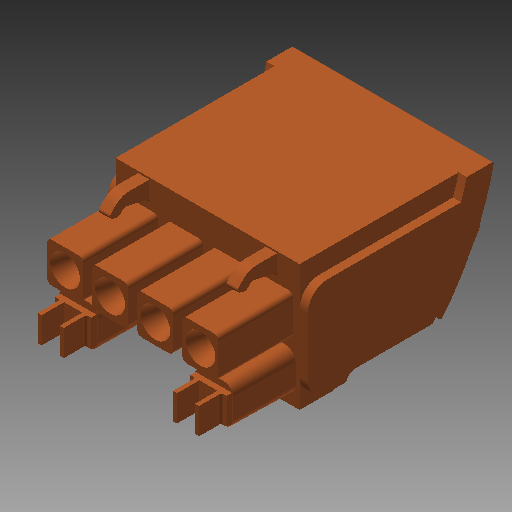
# Autodesk Inventor part: BHZ 5.00/04/90LH BK/OR 1063280000
Saved by Autodesk Inventor 2019.3 (Build 233278000, 278)
## iProperties
Category: PARTsolutions
Company: WEIDMUELLER
Created: 2018-11-15
Part Number: BHZ 5.00/04/90LH BK/OR 1063280000
Material: Generic
Catalog Web Link: www.cadenas.de
Description: BHZ 5.00/90LH-Electronics housings
Vendor: WEIDMUELLER
Document SubType Name: Modeling
Designer: psadmin
Manufacturer: WEIDMUELLER
Mass: 5.49278 g
Surface Area: 32.7214 cm^2
Volume: 5.49278 cm^3
Density: 1 g/cm^3
Appearance: PSOLRGB-219-112-51
PSOL_IDENT_0: {$CADENAS_DATA\23d-libs\weidmueller\elektronikgehaeuse\einbaugehaeuse\ch20m\zubehoer\bhz500_04_90_lh
PSOL_IDENT_1: .prj},213 {VTYP=3D},{NB=BHZ 5.00/04/90LH BK/OR 1063280000},{LINA=BHZ 5.00/04/90LH BK/OR 1063280000},
PSOL_IDENT_2: {NN=BHZ 5.00/90LH},{DATE=31.03.2017 09:22:38},{GEOMDATE=12.03.2014 15:03:00},{VERSION=},{LINEID=10},
PSOL_IDENT_3: {WBVAR=},{WBNUMERIC=}  {NB=BHZ 5.00/04/90LH BK/OR 1063280000},{LINA=BHZ 5.00/04/90LH BK/OR 106328000
PSOL_IDENT_4: 0},{KT=DUMMY},{BEST=1063280000},{BZ=BHZ 5.00/04/90LH BK/OR},{R=5.00},{P=4},{F=schwarz / orange},{FCO
PSOL_IDENT_5: DE=0.86,0.44,0.20,0.00}
NN: BHZ 5.00/90LH
NT: Electronics housings
NB: BHZ 5.00/04/90LH BK/OR 1063280000
NBSYN: $BZ. $BEST.
LINA: BHZ 5.00/04/90LH BK/OR 1063280000
BEST: 1063280000
BZ: BHZ 5.00/04/90LH BK/OR
R: 5
P: 4
F: black / orange
SUPPLIER: WEIDMUELLER
ARTICLENO: BHZ 5.00/04/90LH BK/OR 1063280000
BOMINFO: BHZ 5.00/04/90LH BK/OR 1063280000
CREATOR: CADENAS GmbH
Title: BHZ 5.00/04/90LH BK/OR 1063280000
Author: Cadenas PARTsolutions
Comments: Electronics housings
Autodesk Inventor part; units mm, degrees
sketch "Sketch_1" plane through (-3.6, 0, 0) normal (1, 0, 0) x (0, 0, -1)
  line L0 (0, 5.3) -> (0, -8.7)
  line L1 (0, -8.7) -> (3.6163, -8.7)
  arc A0 (3.6163, -8.7) -> (4.0993, -8.3294) centre (3.6163, -8.2) ccw
  line L2 (4.0993, -8.3294) -> (4.2837, -7.6412)
  arc A1 (5.2496, -6.9) -> (4.2837, -7.6412) centre (5.2496, -7.9) ccw
  line L3 (5.2496, -6.9) -> (13.7691, -6.9)
  arc A2 (13.7691, -6.9) -> (13.9423, -6.8) centre (13.7691, -6.7) ccw
  line L4 (13.9423, -6.8) -> (14.0722, -6.575)
  arc A3 (14.2021, -6.5) -> (14.0722, -6.575) centre (14.2021, -6.65) ccw
  line L5 (14.2021, -6.5) -> (14.2286, -6.5)
  arc A4 (14.4625, -6.635) -> (14.2286, -6.5) centre (14.2286, -6.77) ccw
  line L6 (14.4625, -6.635) -> (14.5371, -6.7642)
  arc A5 (14.5371, -6.7642) -> (14.9821, -6.7975) centre (14.7709, -6.6292) ccw
  arc A6 (14.9821, -6.7975) -> (17.8754, -2.4) centre (-7.6977, 11.2753) ccw
  line L7 (17.8754, -2.4) -> (19.05, -2.4)
  line L8 (19.05, -2.4) -> (19.05, -0.5176)
  arc A7 (19.2612, 0.588) -> (19.05, -0.5176) centre (22.05, -0.5176) ccw
  arc A8 (19.2612, 0.588) -> (20.6278, 5.0571) centre (-7.6977, 11.2753) ccw
  arc A9 (20.6278, 5.0571) -> (20.4324, 5.3) centre (20.4324, 5.1) ccw
  line L9 (20.4324, 5.3) -> (0, 5.3)
  constraints: 20 end point, 20 point on circle, 10 centre point
extrude "Extrusion1" add sketch "Sketch_1" along normal blind 22.2
sketch "Sketch_2" plane through (0, 0, -19.505) normal (0, 0, 1) x (1, 0, 0)
  line L0 (-5, 0.5) -> (20, 0.5)
  line L1 (-5, 0.4) -> (-5, -3)
  line L2 (-5, -3) -> (20, -3)
  line L3 (20, -3) -> (20, 0.45)
  line L4 (20, 0.45) -> (17.4, 0.45)
  line L5 (17.4, 0.45) -> (17.4, 0)
  arc A0 (13.2353, -1.6266) -> (17.4, 0) centre (15, 0) ccw
  arc A1 (13.2353, -1.6266) -> (11.7647, -1.6266) centre (12.5, -2.3043) ccw
  arc A2 (8.2353, -1.6266) -> (11.7647, -1.6266) centre (10, 0) ccw
  arc A3 (8.2353, -1.6266) -> (6.7647, -1.6266) centre (7.5, -2.3043) ccw
  arc A4 (3.2353, -1.6266) -> (6.7647, -1.6266) centre (5, 0) ccw
  arc A5 (3.2353, -1.6266) -> (1.7647, -1.6266) centre (2.5, -2.3043) ccw
  arc A6 (-2.4, 0) -> (1.7647, -1.6266) centre (0, 0) ccw
  line L6 (-2.4, 0) -> (-2.4, 0.4)
  line L7 (-2.4, 0.4) -> (-5, 0.4)
  constraints: 16 end point, 14 point on circle, 7 centre point
revolve "Revolution1" cut sketch "Sketch_2" angle 30 about axis through (-5, 0.5, -19.505) along (-1, 0, 0)
sketch "Sketch_5" plane through (0, 0, 0) normal (1, 0, 0) x (0, 1, 0)
  line L0 (0, -21) -> (0, -16)
  line L1 (0, -16) -> (1.9, -16)
  line L2 (1.9, -16) -> (1.9, -21)
  line L3 (1.9, -21) -> (0, -21)
  line L4 (0, -21) -> (0, -16)
  constraints: 10 end point
revolve "Revolution2" cut sketch "Sketch_5" angle 360 about axis through (0, 0, -21) along (0, 0, -1)
pattern_linear "Rectangular Pattern1" count 4 spacing 5 along (1, 0, 0) of "Revolution2"
sketch "Sketch_7" plane through (0, 0, 0) normal (0, 0, 1) x (1, 0, 0)
  line L0 (-2, 1.7) -> (-2, -1.7)
  arc A0 (-2, -1.7) -> (-1.5, -2.2) centre (-1.5, -1.7) ccw
  line L1 (-1.5, -2.2) -> (1.5, -2.2)
  arc A1 (1.5, -2.2) -> (2, -1.7) centre (1.5, -1.7) ccw
  line L2 (2, -1.7) -> (2, 1.7)
  arc A2 (2, 1.7) -> (1.5, 2.2) centre (1.5, 1.7) ccw
  line L3 (1.5, 2.2) -> (-1.5, 2.2)
  arc A3 (-1.5, 2.2) -> (-2, 1.7) centre (-1.5, 1.7) ccw
  constraints: 8 end point, 8 point on circle, 4 centre point
extrude "Extrusion2" add sketch "Sketch_7" along normal blind 8.3
pattern_linear "Rectangular Pattern2" count 4 spacing 5 along (1, 0, 0) of "Extrusion2"
sketch "Sketch_14" plane through (0, 0, 8.3) normal (0, 0, 1) x (1, 0, 0)
  circle A0 centre (0, 0) radius 1.65
  constraints: 1 centre point
extrude "Extrusion3" cut sketch "Sketch_14" against normal blind 2 draft -15
pattern_linear "Rectangular Pattern3" count 4 spacing 5 along (1, 0, 0) of "Extrusion3"
sketch "Sketch_10" plane through (-3.6, 0, 0) normal (1, 0, 0) x (0, 0, -1)
  line L0 (-2, -9.7) -> (22, -9.7)
  line L1 (22, -9.7) -> (22, -6.9)
  line L2 (22, -6.9) -> (5.8, -6.9)
  arc A0 (5.8, -6.9) -> (5.0615, -7.3923) centre (5.8, -7.7) ccw
  arc A1 (4.6, -7.7) -> (5.0615, -7.3923) centre (4.6, -7.2) ccw
  line L3 (4.6, -7.7) -> (2.2, -7.7)
  arc A2 (0, -5.5) -> (2.2, -7.7) centre (2.2, -5.5) ccw
  line L4 (0, -5.5) -> (0, 1)
  arc A3 (2.2, 3.2) -> (0, 1) centre (2.2, 1) ccw
  line L5 (2.2, 3.2) -> (16.9983, 3.2)
  arc A4 (16.9983, 3.2) -> (17.8445, 6.2) centre (-7.75, 11.8) ccw
  line L6 (17.8445, 6.2) -> (-2, 6.2)
  line L7 (-2, 6.2) -> (-2, -9.7)
  constraints: 16 end point, 10 point on circle, 5 centre point
extrude "Extrusion4" cut sketch "Sketch_10" along normal blind 0.9
sketch "Sketch_28" plane through (18.6, 0, 0) normal (1, 0, 0) x (0, 0, -1)
  line L0 (-2, -9.7) -> (22, -9.7)
  line L1 (22, -9.7) -> (22, -6.9)
  line L2 (22, -6.9) -> (5.8, -6.9)
  arc A0 (5.8, -6.9) -> (5.0615, -7.3923) centre (5.8, -7.7) ccw
  arc A1 (4.6, -7.7) -> (5.0615, -7.3923) centre (4.6, -7.2) ccw
  line L3 (4.6, -7.7) -> (2.2, -7.7)
  arc A2 (0, -5.5) -> (2.2, -7.7) centre (2.2, -5.5) ccw
  line L4 (0, -5.5) -> (0, 1)
  arc A3 (2.2, 3.2) -> (0, 1) centre (2.2, 1) ccw
  line L5 (2.2, 3.2) -> (16.9983, 3.2)
  arc A4 (16.9983, 3.2) -> (17.8445, 6.2) centre (-7.75, 11.8) ccw
  line L6 (17.8445, 6.2) -> (-2, 6.2)
  line L7 (-2, 6.2) -> (-2, -9.7)
  constraints: 16 end point, 10 point on circle, 5 centre point
extrude "Extrusion5" cut sketch "Sketch_28" against normal blind 0.9
sketch "Sketch_12" plane through (0, -8, 0) normal (0, 1, 0) x (1, 0, 0)
  line L0 (-2.1, 4.3) -> (2.1, 4.3)
  line L1 (2.1, 4.3) -> (2.1, 10.4)
  line L2 (2.1, 10.4) -> (-2.1, 10.4)
  line L3 (-2.1, 10.4) -> (-2.1, 4.3)
  constraints: 8 end point
extrude "Extrusion6" cut sketch "Sketch_12" along normal blind 4.5 draft -5
pattern_linear "Rectangular Pattern4" count 4 spacing 5 along (1, 0, 0) of "Extrusion6"
sketch "Sketch_16" plane through (0, 0, 0) normal (0, 0, 1) x (1, 0, 0)
  line L0 (-2.25, -4.35) -> (-2.25, -6.55)
  arc A0 (-2.25, -6.55) -> (-1.1, -7.7) centre (-1.1, -6.55) ccw
  line L1 (-1.1, -7.7) -> (1.1, -7.7)
  arc A1 (1.1, -7.7) -> (2.25, -6.55) centre (1.1, -6.55) ccw
  line L2 (2.25, -6.55) -> (2.25, -4.35)
  arc A2 (2.25, -4.35) -> (1.1, -3.2) centre (1.1, -4.35) ccw
  line L3 (1.1, -3.2) -> (-1.1, -3.2)
  arc A3 (-1.1, -3.2) -> (-2.25, -4.35) centre (-1.1, -4.35) ccw
  constraints: 8 end point, 8 point on circle, 4 centre point
extrude "Extrusion7" add sketch "Sketch_16" along normal blind 6.8 draft -0.5
sketch "Sketch_17" plane through (0, 0, 0) normal (0, 0, 1) x (1, 0, 0)
  line L0 (12.75, -4.35) -> (12.75, -6.55)
  arc A0 (12.75, -6.55) -> (13.9, -7.7) centre (13.9, -6.55) ccw
  line L1 (13.9, -7.7) -> (16.1, -7.7)
  arc A1 (16.1, -7.7) -> (17.25, -6.55) centre (16.1, -6.55) ccw
  line L2 (17.25, -6.55) -> (17.25, -4.35)
  arc A2 (17.25, -4.35) -> (16.1, -3.2) centre (16.1, -4.35) ccw
  line L3 (16.1, -3.2) -> (13.9, -3.2)
  arc A3 (13.9, -3.2) -> (12.75, -4.35) centre (13.9, -4.35) ccw
  constraints: 8 end point, 8 point on circle, 4 centre point
extrude "Extrusion8" add sketch "Sketch_17" along normal blind 6.8 draft -1
sketch "Sketch_18" plane through (0, -5.45, 0) normal (0, 1, 0) x (1, 0, 0)
  line L0 (-2, -7.4) -> (-1.65, -7.4)
  arc A0 (-1.45, -7.6) -> (-1.65, -7.4) centre (-1.65, -7.6) ccw
  line L1 (-1.45, -7.6) -> (-1.45, -9.9)
  line L2 (-1.45, -9.9) -> (-1, -9.9)
  line L3 (-1, -9.9) -> (-1, -7.4)
  line L4 (-1, -7.4) -> (1, -7.4)
  line L5 (1, -7.4) -> (1, -9.9)
  line L6 (1, -9.9) -> (1.45, -9.9)
  line L7 (1.45, -9.9) -> (1.45, -7.6)
  arc A1 (1.65, -7.4) -> (1.45, -7.6) centre (1.65, -7.6) ccw
  line L8 (1.65, -7.4) -> (2, -7.4)
  line L9 (2, -7.4) -> (2, -6.8)
  line L10 (2, -6.8) -> (-2, -6.8)
  line L11 (-2, -6.8) -> (-2, -7.4)
  constraints: 24 end point, 4 point on circle, 2 centre point
extrude "Extrusion9" add sketch "Sketch_18" along normal mid plane 2.9
sketch "Sketch_19" plane through (0, -5.45, 0) normal (0, 1, 0) x (1, 0, 0)
  line L0 (13, -7.4) -> (13.35, -7.4)
  arc A0 (13.55, -7.6) -> (13.35, -7.4) centre (13.35, -7.6) ccw
  line L1 (13.55, -7.6) -> (13.55, -9.9)
  line L2 (13.55, -9.9) -> (14, -9.9)
  line L3 (14, -9.9) -> (14, -7.4)
  line L4 (14, -7.4) -> (16, -7.4)
  line L5 (16, -7.4) -> (16, -9.9)
  line L6 (16, -9.9) -> (16.45, -9.9)
  line L7 (16.45, -9.9) -> (16.45, -7.6)
  arc A1 (16.65, -7.4) -> (16.45, -7.6) centre (16.65, -7.6) ccw
  line L8 (16.65, -7.4) -> (17, -7.4)
  line L9 (17, -7.4) -> (17, -6.8)
  line L10 (17, -6.8) -> (13, -6.8)
  line L11 (13, -6.8) -> (13, -7.4)
  constraints: 24 end point, 4 point on circle, 2 centre point
extrude "Extrusion10" add sketch "Sketch_19" along normal mid plane 2.9
sketch "Sketch_21" plane through (0, -4.4, 0) normal (0, 1, 0) x (1, 0, 0)
  line L0 (3.5, 18.5) -> (3.5, 16)
  line L1 (3.5, 16) -> (11.5, 16)
  line L2 (11.5, 16) -> (11.5, 18.5)
  arc A0 (11.5, 18.5) -> (10, 20) centre (10, 18.5) ccw
  line L3 (10, 20) -> (5, 20)
  arc A1 (5, 20) -> (3.5, 18.5) centre (5, 18.5) ccw
  constraints: 8 end point, 4 point on circle, 2 centre point
extrude "Extrusion11" add sketch "Sketch_21" along normal blind 0.8
sketch "Sketch_26" plane through (-0.2, 0, 0) normal (1, 0, 0) x (0, 0, -1)
  arc A0 (-4.3047, 3.9096) -> (-4.1952, 3.4191) centre (-4.09, 3.7) ccw
  line L0 (-4.1952, 3.4191) -> (-3.7754, 3.2618)
  arc A1 (-3.7754, 3.2618) -> (-3.2404, 3.3826) centre (-3.6, 3.73) ccw
  line L1 (-3.2404, 3.3826) -> (-2.9846, 3.6474)
  arc A2 (-2.5212, 3.7891) -> (-2.9846, 3.6474) centre (-2.625, 3.3) ccw
  line L2 (-2.5212, 3.7891) -> (-0.3122, 3.3203)
  arc A3 (0, 2.93) -> (-0.3122, 3.3203) centre (-0.4, 2.93) ccw
  line L3 (0, 2.93) -> (0, 5.1)
  line L4 (0, 5.1) -> (-2.3, 5.1)
  arc A4 (-2.3, 5.1) -> (-3.7311, 4.4971) centre (-2.3, 3.1) ccw
  line L5 (-3.7311, 4.4971) -> (-4.3047, 3.9096)
  constraints: 12 end point, 10 point on circle, 5 centre point
extrude "Extrusion12" add sketch "Sketch_26" along normal blind 1.25
sketch "Sketch_27" plane through (15.2, 0, 0) normal (1, 0, 0) x (0, 0, -1)
  arc A0 (-4.3047, 3.9096) -> (-4.1952, 3.4191) centre (-4.09, 3.7) ccw
  line L0 (-4.1952, 3.4191) -> (-3.7754, 3.2618)
  arc A1 (-3.7754, 3.2618) -> (-3.2404, 3.3826) centre (-3.6, 3.73) ccw
  line L1 (-3.2404, 3.3826) -> (-2.9846, 3.6474)
  arc A2 (-2.5212, 3.7891) -> (-2.9846, 3.6474) centre (-2.625, 3.3) ccw
  line L2 (-2.5212, 3.7891) -> (-0.3122, 3.3203)
  arc A3 (0, 2.93) -> (-0.3122, 3.3203) centre (-0.4, 2.93) ccw
  line L3 (0, 2.93) -> (0, 5.1)
  line L4 (0, 5.1) -> (-2.3, 5.1)
  arc A4 (-2.3, 5.1) -> (-3.7311, 4.4971) centre (-2.3, 3.1) ccw
  line L5 (-3.7311, 4.4971) -> (-4.3047, 3.9096)
  constraints: 12 end point, 10 point on circle, 5 centre point
extrude "Extrusion13" add sketch "Sketch_27" against normal blind 1.25
ref_plane "mitMark_BHZ_XY" through (7.5, -4.4, -16.635) normal (0, 0, 1) x (1, 0, 0)
ref_plane "mitMark_BHZ_YZ" through (7.5, -4.4, -16.635) normal (1, 0, 0) x (0, 1, 0)
ref_plane "mitMark_BHZ_ZX" through (7.5, -4.4, -16.635) normal (0, 1, 0) x (0, 0, 1)
ref_plane "mitMark_BHZ_2p_XY" through (2.5, -4.4, -16.635) normal (0, 0, 1) x (1, 0, 0)
ref_plane "mitMark_BHZ_2p_YZ" through (2.5, -4.4, -16.635) normal (1, 0, 0) x (0, 1, 0)
ref_plane "mitMark_BHZ_2p_ZX" through (2.5, -4.4, -16.635) normal (0, 1, 0) x (0, 0, 1)
ref_plane "mitMark_BHZ_3p_XY" through (5, -4.4, -16.635) normal (0, 0, 1) x (1, 0, 0)
ref_plane "mitMark_BHZ_3p_YZ" through (5, -4.4, -16.635) normal (1, 0, 0) x (0, 1, 0)
ref_plane "mitMark_BHZ_3p_ZX" through (5, -4.4, -16.635) normal (0, 1, 0) x (0, 0, 1)
ref_plane "mitSHL_XY" through (0, 0, 0) normal (0, 0, -1) x (1, 0, 0)
ref_plane "mitSHL_YZ" through (0, 0, 0) normal (1, 0, 0) x (0, -1, 0)
ref_plane "mitSHL_ZX" through (0, 0, 0) normal (0, -1, 0) x (0, 0, -1)
ref_plane "mitSHL_li_2_XY" through (5, 0, 0) normal (0, 0, -1) x (1, 0, 0)
ref_plane "mitSHL_li_2_YZ" through (5, 0, 0) normal (1, 0, 0) x (0, -1, 0)
ref_plane "mitSHL_li_2_ZX" through (5, 0, 0) normal (0, -1, 0) x (0, 0, -1)
ref_plane "mitSHL_li_3_XY" through (10, 0, 0) normal (0, 0, -1) x (1, 0, 0)
ref_plane "mitSHL_li_3_YZ" through (10, 0, 0) normal (1, 0, 0) x (0, -1, 0)
ref_plane "mitSHL_li_3_ZX" through (10, 0, 0) normal (0, -1, 0) x (0, 0, -1)
ref_plane "mitSHL_li_4_XY" through (15, 0, 0) normal (0, 0, -1) x (1, 0, 0)
ref_plane "mitSHL_li_4_YZ" through (15, 0, 0) normal (1, 0, 0) x (0, -1, 0)
ref_plane "mitSHL_li_4_ZX" through (15, 0, 0) normal (0, -1, 0) x (0, 0, -1)
body "Solid1"
